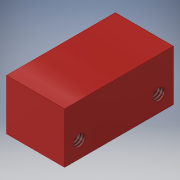
# Autodesk Inventor part: CHA_013_2inCrossPlug
Saved by Autodesk Inventor 2018.3 (Build 223284000, 284)
## iProperties
Created: 2018-01-20
Part Number: CHA_013_2inCrossPlug
Material: Aluminum 6061
Document SubType Name: Modeling
Designer: irodr
Density: 2.7 g/cm^3
Appearance: Orange-Red
Mass: 69.9197 g
Surface Area: 63.8197 cm^2
Volume: 25.8962 cm^3
Author: irodr
Autodesk Inventor part; units mm, degrees
ref_plane "YZ Plane" through (0, 0, 0) normal (1, 0, 0) x (0, 1, 0)
ref_plane "XZ Plane" through (0, 0, 0) normal (0, 1, 0) x (-1, 0, 0)
ref_plane "XY Plane" through (0, 0, 0) normal (0, 0, 1) x (1, 0, 0)
sketch "Sketch1" plane through (0, 0, 0) normal (0, 0, 1) x (1, 0, 0)
  line L0 (0, 0) -> (25.4, 0)
  line L1 (25.4, 0) -> (25.4, 22.225)
  line L2 (25.4, 22.225) -> (0, 22.225)
  line L3 (0, 22.225) -> (0, 0)
  dimension "d0" = 25.4
  dimension "d1" = 22.225
  constraints: 8 end point, 2 parallel, 1 horizontal, 1 perpendicular
  measures "d0" distance of L2.end L1.end
  measures "d1" distance of L1.end L0.end
extrude "Extrusion1" add sketch "Sketch1" along normal blind 47.625
sketch "Sketch3" plane through (0, 0, 0) normal (-1, 0, 0) x (0, 0, 1)
  line L0 (0, 22.225) -> (0, 0) projected
  line L1 (0, 0) -> (47.625, 0) projected
  line L2 (47.625, 22.225) -> (47.625, 0) projected
  line L3 (0, 22.225) -> (47.625, 22.225) projected
  point P0 (41.275, 7.112)
  point P1 (6.35, 7.112)
  dimension "d15" = 7.112
  dimension "d16" = 7.112
  dimension "d17" = 34.925
  dimension "d18" = 6.35
  measures "d15" distance from line of point (41.275, 7.112) L1
  measures "d16" distance from line of L1 point (6.35, 7.112)
  measures "d17" distance of point (41.275, 7.112) point (6.35, 7.112)
  measures "d18" distance from line of L2 point (41.275, 7.112)
hole "Hole2" at (0, 7.112, 41.275) at (0, 7.112, 6.35) direction (1, 0, 0) diameter 4.9784 end through all thread size "1/4-20 UNC" class "2B" standard "ANSI Unified Screw Threads"
body "Solid1"
